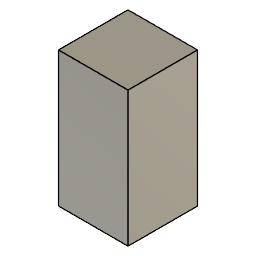
Final Design - Clawser Cabinet Model (Autodesk Fusion 360 archive; units mm, degrees)
design "Stopper Test"
Autodesk Fusion 360 part; units mm, degrees
sketch "Sketch1" plane through (0, 0, 0) normal (0, 0, 1) x (1, 0, 0)
  line L0 (9, 9) -> (-9, 9)
  line L1 (-9, 9) -> (-9, -9)
  line L2 (-9, -9) -> (9, -9)
  line L3 (9, -9) -> (9, 9)
  line L4 (9, 9) -> (-9, -9) construction
  line L5 (-9, 9) -> (9, -9) construction
  dimension "d1" = 18
  dimension "d2" = 18
  constraint horizontal L0
  constraint perpendicular L0 L1
  constraint parallel L0 L2
  constraint parallel L1 L3
  constraint coincident L4 origin
  constraint coincident L5 origin
  measures "d1" distance of L1.end L2.end
  measures "d2" distance of L0.end L1.end
extrude "Extrude1" add sketch "Sketch1" along normal blind 35

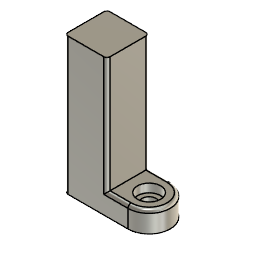
design "Switch Endstopper"
Autodesk Fusion 360 part; units mm, degrees
sketch "Sketch1" plane through (0, 0, 0) normal (0, 0, 1) x (1, 0, 0)
  line L0 (-10, -10) -> (10, -10)
  line L1 (10, -10) -> (10, 10)
  line L2 (10, 10) -> (-10, 10)
  line L3 (-10, 10) -> (-10, -10)
  line L4 (-10, -10) -> (10, 10) construction
  line L5 (10, -10) -> (-10, 10) construction
  dimension "d1" = 20
  dimension "d2" = 20
  constraint horizontal L0
  constraint perpendicular L0 L1
  constraint parallel L0 L2
  constraint parallel L1 L3
  constraint coincident L4 origin
  constraint coincident L5 origin
  measures "d1" distance of L1.end L2.end
  measures "d2" distance of L0.end L1.end
extrude "Extrude1" add sketch "Sketch1" along normal blind 65
sketch "Sketch2" plane through (0, 0, 0) normal (0, 0, -1) x (1, 0, 0)
  line L0 (-10, 10) -> (-10, -10)
  line L1 (-10, -10) -> (10, -10)
  line L2 (10, -10) -> (10, 10)
  line L3 (10, 10) -> (-10, 10)
  line L4 (10, 10) -> (10, -10)
  line L5 (10, -10) -> (10, 10)
  line L6 (10, 10) -> (30, 10) construction
  line L7 (30, 10) -> (30, -10) construction
  line L8 (30, -10) -> (10, -10) construction
  arc A0 (20, -10) -> (20, 10) centre (20, 0) ccw
  line L9 (20, -10) -> (10, -10) construction
  line L10 (10, -10) -> (10, 10) construction
  line L11 (20, -10) -> (10, -10)
  line L12 (20, 10) -> (10, 10)
  point P0 (10, -10)
  point P1 (10, 10)
  dimension "d5" = 20
  constraint perpendicular L5 L6
  constraint parallel L5 L7
  constraint parallel L6 L8
  constraint coincident P1 L2.end
  constraint perpendicular L3 L5
  constraint coincident P0 L1.end
  constraint tangent L7 A0
  constraint midpoint L8 A0.start
  constraint midpoint L6 A0.end
  measures "d5" distance of P0 L7.end
extrude "Extrude2" add sketch "Sketch2" against normal blind 10 contours L2 L4 L5 A0 L11 L12
sketch "Sketch4" plane through (0, 0, 10) normal (0, 0, 1) x (-1, 0, 0)
  arc A0 (-20, 10) -> (-20, -10) centre (-20, 0) ccw
  line L0 (-20, -10) -> (-10, -10)
  line L1 (-10, -10) -> (-10, 10)
  line L2 (-10, 10) -> (-20, 10)
  line L3 (-20, 10) -> (-20, -10) construction
  point P0 (-20, 10)
  point P1 (-20, -10)
  constraint coincident P0 A0.start
  constraint coincident P1 A0.end
hole "Hole1" at (20, 0, 10) direction (0, 0, -1) diameter 6.5 depth 10 tip angle 180 counterbore diameter 11 counterbore depth 4
sketch "Sketch5" plane through (0, 0, 0) normal (0, 0, -1) x (1, 0, 0)
  circle A0 centre (20, 0) radius 3.25
  line L0 (-10, 10) -> (-10, -10)
  line L1 (-10, -10) -> (20, -10)
  arc A1 (20, -10) -> (20, 10) centre (20, 0) ccw
  line L2 (20, 10) -> (-10, 10)
  line L3 (6, 3.8) -> (-6, 3.8)
  line L4 (-6, 3.8) -> (-6, -3.8)
  line L5 (-6, -3.8) -> (6, -3.8)
  line L6 (6, -3.8) -> (6, 3.8)
  line L7 (6, 3.8) -> (-6, -3.8) construction
  line L8 (-6, 3.8) -> (6, -3.8) construction
  dimension "d13" = 12
  dimension "d14" = 7.6
  constraint horizontal L3
  constraint perpendicular L3 L4
  constraint parallel L3 L5
  constraint parallel L4 L6
  constraint coincident L7 origin
  constraint coincident L8 origin
  measures "d13" distance of L4.end L5.end
  measures "d14" distance of L3.end L4.end
extrude "Extrude3" add sketch "Sketch5" along normal blind 2 contours L3 L4 L5 L6
fillet "Fillet1" radius 1.5 11 edges at (-10, 10, 32.5) (-10, -10, 32.5) (10, -10, 37.5) (15, -10, 10) (30, 0, 10) (15, 10, 10) (10, 10, 37.5) (6, 3.8, -1) (6, -3.8, -1) (-6, -3.8, -1) (-6, 3.8, -1)
